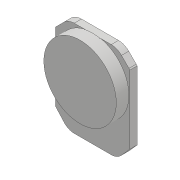
# Autodesk Inventor part: table
Saved by Autodesk Inventor 2018 (Build 220112000, 112)
## iProperties
Created: 2018-02-04
Part Number: table
Material: Generic
Document SubType Name: Modeling
Designer: Clevo
Density: 1 g/cm^3
Appearance: Default
Author: Clevo
Autodesk Inventor part; units mm, degrees
ref_plane "YZ Plane" through (0, 0, 0) normal (1, 0, 0) x (0, 1, 0)
ref_plane "XZ Plane" through (0, 0, 0) normal (0, 1, 0) x (-1, 0, 0)
ref_plane "XY Plane" through (0, 0, 0) normal (0, 0, 1) x (1, 0, 0)
sketch "Sketch1" plane through (0, 0, 0) normal (0, 1, 0) x (-1, 0, 0)
  circle A0 centre (0, 0) radius 20
  dimension "d0" = 40
  constraints: 1 centre point, 1 coincident
  measures "d0" diameter of A0
extrude "Extrusion1" add sketch "Sketch1" along normal blind 7
sketch "Sketch2" plane through (0, 7, 0) normal (0, 1, 0) x (1, 0, 0)
  circle A0 centre (0, 0) radius 40.2
  dimension "d3" = 80.4
  constraints: 1 centre point, 1 coincident
  measures "d3" diameter of A0
extrude "Extrusion2" add sketch "Sketch2" along normal blind 4
sketch "Sketch10" plane through (0, 11, 0) normal (0, 1, 0) x (1, 0, 0)
  circle A0 centre (0, 0) radius 40.2 projected
  circle A1 centre (12, 8) radius 1.6 projected
  circle A2 centre (-12, 8) radius 1.6 projected
  circle A3 centre (-12, -9) radius 1.6 projected
  circle A4 centre (12, -9) radius 1.6 projected
  ellipse E0 centre (10.2363, 24.2903) end of major axis (10.2363, 33.2346) minor radius 8 (15.8931, 30.6149) -> (10.2363, 33.2346) ccw projected
  line L0 (20.55, 25.4083) -> (15.8931, 30.6149) projected
  line L1 (20.55, 25.4083) -> (20.55, -12.4582) projected
  ellipse E1 centre (16.4789, -9.4868) end of major axis (22.6027, -3.3631) minor radius 5 (20.0145, -13.0223) -> (20.55, -12.4582) ccw projected
  line L2 (15.8931, -17.1436) -> (20.0145, -13.0223) projected
  arc A5 (10.2363, -19.4868) -> (15.8931, -17.1436) centre (10.2363, -11.4868) ccw projected
  line L3 (-10.2363, -19.4868) -> (10.2363, -19.4868) projected
  arc A6 (-15.8931, -17.1436) -> (-10.2363, -19.4868) centre (-10.2363, -11.4868) ccw projected
  line L4 (-20.0145, -13.0223) -> (-15.8931, -17.1436) projected
  ellipse E2 centre (-16.4789, -9.4868) end of major axis (-22.6027, -3.3631) minor radius 5 (-20.55, -12.4582) -> (-20.0145, -13.0223) ccw projected
  line L5 (-20.55, -12.4582) -> (-20.55, 25.4083) projected
  line L6 (-15.8931, 30.6149) -> (-20.55, 25.4083) projected
  ellipse E3 centre (-10.2363, 24.2903) end of major axis (-10.2363, 33.2346) minor radius 8 (-10.2363, 33.2346) -> (-15.8931, 30.6149) ccw projected
  line L7 (-10.2363, 33.2346) -> (10.2363, 33.2346) projected
  constraints: 4 other
ref_plane "Work Plane1" through (-40.2, 6.8, -40.2) normal (0, 1, 0) x (0, 0, 1)
extrude "Extrusion7" cut sketch "Sketch10" against normal up to surface (4.2 mm away) contours A0
body "Solid1"
